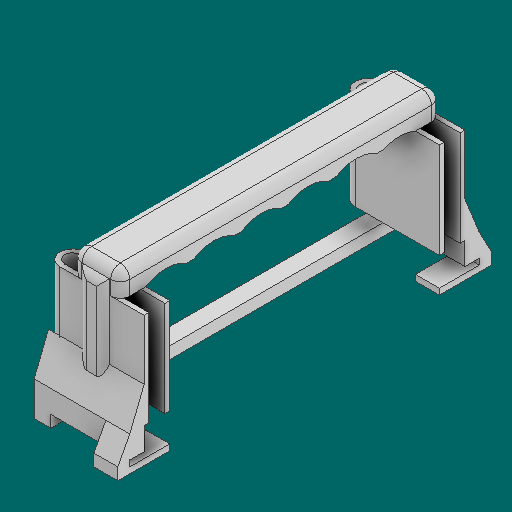
# Autodesk Inventor part: lab2
Saved by Autodesk Inventor 2026.1 (Build 301233000, 233)
## iProperties
Created: 2025-10-02
Part Number: lab2
Material: Genérico
Document SubType Name: Modeling
Designer: norbe
Density: 1 g/cm^3
Appearance: Valor por defecto
Author: norbe
Autodesk Inventor part; units mm, degrees
ref_plane "YZ Plane" through (0, 0, 0) normal (1, 0, 0) x (0, 1, 0)
ref_plane "XZ Plane" through (0, 0, 0) normal (0, 1, 0) x (-1, 0, 0)
sketch "Boceto1" plane through (0, 0, 0) normal (0, 1, 0) x (-1, 0, 0)
  line L0 (0, 0) -> (70.5, 0)
  line L1 (70.5, 0) -> (70.5, -135)
  line L2 (70.5, -135) -> (0, -135)
  line L3 (0, -135) -> (0, 0)
  line L4 (35.25, -64.3132) -> (35.25, -123.8882)
  line L5 (35.25, -125.8882) -> (35.25, -132.5882)
  arc A0 (35.25, -132.5882) -> (35.25, -125.8882) centre (35.25, -129.2382) ccw
  line L6 (0, -67.5) -> (7.0984, -67.5)
  arc A1 (35.25, -134.5882) -> (35.25, -123.8882) centre (35.25, -129.2382) ccw
  line L7 (35.25, -123.8882) -> (0, -123.8882)
  line L8 (35.25, -134.5882) -> (0, -134.5882)
  line L9 (35.25, -125.8882) -> (0, -125.8882)
  line L10 (35.25, -132.5882) -> (0, -132.5882)
  arc A2 (35.25, -11.1118) -> (35.25, -0.4118) centre (35.25, -5.7618) ccw
  line L11 (35.25, -11.1118) -> (0, -11.1118)
  line L12 (35.25, -0.4118) -> (0, -0.4118)
  arc A3 (35.25, -9.1118) -> (35.25, -2.4118) centre (35.25, -5.7618) ccw
  line L13 (35.25, -9.1118) -> (0, -9.1118)
  line L14 (35.25, -2.4118) -> (0, -2.4118)
  dimension "d0" = 70.5
  dimension "d1" = 135
  dimension "d2" = 61.575
  dimension "d3" = 6.7
  dimension "d4" = 67.5
  dimension "d5" = 2
  constraints: 30 end point, 10 symmetric about line, 8 point on circle, 4 centre point, 4 point on line, 3 horizontal, 3 parallel, 3 perpendicular, 2 midpoint, 2 tangent, 2 vertical, 2 other
  measures "d0" distance of L1.end L2.end
  measures "d1" distance of L0.end L1.end
  measures "d2" distance of L4.start L5.start
  measures "d3" distance of L5.end L5.start
  measures "d4" distance between parallel lines of L2 L6
  measures "d5" radial gap between concentric circles of A0 A1
extrude "Extrusión1" add sketch "Boceto1" along normal blind 40 contours L12 A2 L11 L3 L13 A3 L14 | L3 L10 A0 L9 L7 A1 L8
sketch "Boceto2" plane through (0, 0, -0.4118) normal (1, 0, 0) x (0, 0, -1)
  line L0 (0, 0) -> (2, 0) projected
  line L1 (2, 0) -> (2, 40) projected
  line L2 (0, 40) -> (2, 40) projected
  line L3 (0, 0) -> (0, 40) projected
  line L4 (132.1764, 0) -> (134.1764, 0) projected
  line L5 (134.1764, 0) -> (134.1764, 40) projected
  line L6 (132.1764, 40) -> (134.1764, 40) projected
  line L7 (132.1764, 0) -> (132.1764, 40) projected
  line L8 (0, 0) -> (134.1764, 0)
  line L9 (134.1764, 0) -> (134.1764, -9.4)
  line L10 (134.1764, -9.4) -> (0, -9.4)
  line L11 (0, -9.4) -> (0, 0)
  line L12 (134.1764, -9.4) -> (-1.655, -9.4)
  line L13 (-1.655, -9.4) -> (-1.655, -12.4)
  line L14 (-1.655, -12.4) -> (134.1764, -12.4)
  line L15 (134.1764, -12.4) -> (134.1764, -9.4)
  line L16 (134.1764, 0) -> (134.1764, 15)
  line L17 (134.1764, 0) -> (134.1764, 40) projected
  line L18 (134.1764, 0) -> (149.1764, 0) construction
  line L19 (134.1764, -9.4) -> (140.1764, -9.4)
  line L20 (140.1764, -9.4) -> (140.1764, 0)
  line L21 (134.1764, 15) -> (140.1764, 0)
  line L22 (67.0882, 0) -> (67.0882, 3.7714)
  line L23 (0, 0) -> (0, -9.4)
  line L24 (0, 0) -> (0, 15)
  line L25 (0, -9.4) -> (-6, -9.4)
  line L26 (-6, -9.4) -> (-6, 0)
  line L27 (0, 15) -> (-6, 0)
  point P0 (-0.4118, 0)
  point P1 (134.1764, 0)
  point P2 (0, -9.4)
  point P3 (0, -9.4)
  dimension "d8" = 9.4
  dimension "d9" = 3
  dimension "d19" = 15
  dimension "d20" = 90
  dimension "d21" = 6
  constraints: 38 end point, 4 horizontal, 4 parallel, 4 perpendicular, 4 symmetric about line, 1 collinear, 1 midpoint, 1 point on line, 1 vertical
  measures "d8" distance of L8.end L9.end
  measures "d9" distance of L13.end L12.end
  measures "d19" distance of L8.end L16.end
  measures "d20" angle of L18 L16
  measures "d21" distance of L9.end L19.end
extrude "Extrusión2" add sketch "Boceto2" against normal blind 40 contours L11 L12 L25 L26 L27 L3 | L0 L8 L4 L9 L10 L11 | L9 L5 L21 L20 L19
extrude "Extrusión3" add sketch "Boceto2" against normal blind 5 contours L10 L15 L14 L13 L12
sketch "Boceto4" plane through (-40, 0, -0.4118) normal (-1, 0, 0) x (0, 0, 1)
  line L0 (-134.1764, 15) -> (-140.1764, 0) projected
  line L1 (-140.1764, 0) -> (-140.1764, -9.4) projected
  line L2 (-140.1764, -9.4) -> (6, -9.4) projected
  line L3 (6, -9.4) -> (6, 0) projected
  line L4 (6, 0) -> (0, 15) projected
  line L5 (0, 15) -> (0, 0) projected
  line L6 (0, 0) -> (-2.8883, 0) projected
  line L7 (-7.8117, 0) -> (-2.8883, 0) projected
  line L8 (-7.8117, 0) -> (-126.3647, 0) projected
  line L9 (-131.2881, 0) -> (-126.3647, 0) projected
  line L10 (-131.2881, 0) -> (-134.1764, 0) projected
  line L11 (-134.1764, 0) -> (-134.1764, 15) projected
  line L12 (-140.1764, -9.4) -> (6, -9.4)
  line L13 (6, -9.4) -> (6, -14.4)
  line L14 (6, -14.4) -> (-140.1764, -14.4)
  line L15 (-140.1764, -14.4) -> (-140.1764, -9.4)
  line L16 (0, 0) -> (0, -9.4)
  line L17 (-134.1764, 0) -> (-134.1764, -9.4)
  point P0 (0.4118, 0)
  dimension "d22" = 5
  constraints: 12 end point, 3 perpendicular, 2 parallel, 2 point on line, 1 horizontal
  measures "d22" distance of L12.end L13.end
extrude "Extrusión4" cut sketch "Boceto4" against normal blind 40 contours L10 L9 L8 L7 L6 L16 L2 L17 | L2 L13 L14 L15
extrude "Extrusión5" add sketch "Boceto4" against normal blind 7 contours L2 L13 L14 L15
sketch "Boceto5" plane through (0, 0, -2.4118) normal (1, 0, 0) x (0, 0, -1)
  line L0 (-2, 40) -> (132.1764, 40)
  line L1 (132.1764, 40) -> (132.1764, 46)
  line L2 (128.1764, 50) -> (2, 50)
  line L3 (-2, 46) -> (-2, 40)
  arc A0 (25.7, 40) -> (8.7, 40) centre (17.2, 26.4446) ccw
  arc A1 (25.7, 40) -> (28.7, 40) centre (27.2, 44.7697) ccw
  line L4 (28.7, 40) -> (28.7, 41.5335)
  arc A2 (45.7, 40) -> (28.7, 40) centre (37.2, 26.4446) ccw
  arc A3 (45.7, 40) -> (48.7, 40) centre (47.2, 44.5587) ccw
  line L5 (48.7, 40) -> (48.7, 40.7668)
  arc A4 (65.7, 40) -> (48.7, 40) centre (57.2, 26.4446) ccw
  arc A5 (65.7, 40) -> (68.1808, 40) centre (66.9404, 43.0685) ccw
  arc A6 (85.1808, 40) -> (68.1808, 40) centre (76.6808, 26.4446) ccw
  arc A7 (85.1808, 40) -> (88.1808, 40) centre (86.6808, 44.5366) ccw
  arc A8 (105.1808, 40) -> (88.1808, 40) centre (96.6808, 26.4446) ccw
  arc A9 (105.1808, 40) -> (108.1808, 40) centre (106.6808, 42.3921) ccw
  arc A10 (121.4764, 40) -> (108.1808, 40) centre (114.8286, 25.4464) ccw
  arc A11 (2, 50) -> (-2, 46) centre (2, 46) ccw
  arc A12 (132.1764, 46) -> (128.1764, 50) centre (128.1764, 46) ccw
  point P0 (-2.4118, 0)
  point P1 (132.1764, 50)
  dimension "d27" = 10
  dimension "d28" = 17
  dimension "d29" = 16
  dimension "d30" = 5
  dimension "d31" = 3
  dimension "d32" = 17
  dimension "d33" = 16
  dimension "d39" = 3
  dimension "d40" = 17
  dimension "d41" = 16
  dimension "d42" = 17
  dimension "d43" = 16
  dimension "d44" = 3
  dimension "d45" = 17
  dimension "d46" = 16
  dimension "d47" = 3
  dimension "d48" = 16
  dimension "d49" = 4
  constraints: 26 point on circle, 13 centre point, 10 end point, 5 tangent, 3 vertical, 2 point on line, 1 coincident, 1 equal radius, 1 horizontal, 1 parallel, 13 other
  measures "d27" distance of point (132.176, 50) L1.start
  measures "d28" distance of A0.end A0.start
  measures "d29" radius of A0
  measures "d30" radius of A1
  measures "d31" distance of A0.start L4.start
  measures "d32" distance of L4.start A2.start
  measures "d33" radius of A2
  measures "d39" distance of A2.start L5.start
  measures "d40" distance of L5.start A4.start
  measures "d41" radius of A4
  measures "d42" distance of A5.end A6.start
  measures "d43" radius of A6
  measures "d44" distance of A6.start A7.end
  measures "d45" distance of A7.end A8.start
  measures "d46" radius of A8
  measures "d47" distance of A8.start A9.end
  measures "d48" radius of A10
  measures "d49" radius of A11
extrude "Extrusión6" add sketch "Boceto5" against normal blind 30 contours L3 A11 L2 A12 L1 L0 A10 A8 A6 A4 A2 A0
sketch "Boceto6" plane through (0, -9.4, -140.5882) normal (1, 0, 0) x (0, 0, -1)
  line L0 (-131.4764, 9.4) -> (-129.4764, 9.4) projected
  line L1 (-129.4764, 9.4) -> (-129.4764, 49.4) projected
  arc A0 (-112.4764, 49.4) -> (-129.4764, 49.4) centre (-120.9764, 35.8446) ccw projected
  line L2 (-112.4764, 49.4) -> (-109.4764, 49.4) projected
  arc A1 (-92.4764, 49.4) -> (-109.4764, 49.4) centre (-100.9764, 35.8446) ccw projected
  line L3 (-92.4764, 49.4) -> (-89.4764, 49.4) projected
  arc A2 (-72.4764, 49.4) -> (-89.4764, 49.4) centre (-80.9764, 35.8446) ccw projected
  line L4 (-72.4764, 49.4) -> (-69.9956, 49.4) projected
  arc A3 (-52.9956, 49.4) -> (-69.9956, 49.4) centre (-61.4956, 35.8446) ccw projected
  line L5 (-52.9956, 49.4) -> (-49.9956, 49.4) projected
  arc A4 (-32.9956, 49.4) -> (-49.9956, 49.4) centre (-41.4956, 35.8446) ccw projected
  line L6 (-32.9956, 49.4) -> (-29.9956, 49.4) projected
  arc A5 (-16.7, 49.4) -> (-29.9956, 49.4) centre (-23.3478, 34.8464) ccw projected
  line L7 (-16.7, 9.4) -> (-16.7, 49.4) projected
  line L8 (-16.7, 9.4) -> (-14.7, 9.4) projected
  line L9 (-14.7, 9.4) -> (-14.7, 49.4) projected
  line L10 (-14.7, 49.4) -> (-8, 49.4) projected
  line L11 (-8, 9.4) -> (-8, 49.4) projected
  line L12 (-8, 9.4) -> (-6, 9.4) projected
  line L13 (-6, 9.4) -> (-6, 0) projected
  line L14 (-6, 0) -> (0, 0) projected
  line L15 (0, 0) -> (0, 9.4) projected
  line L16 (0, 9.4) -> (-6, 24.4) projected
  line L17 (-6, 24.4) -> (-6, 55.4) projected
  arc A6 (-6, 55.4) -> (-10, 59.4) centre (-10, 55.4) ccw projected
  line L18 (-10, 59.4) -> (-136.1764, 59.4) projected
  arc A7 (-136.1764, 59.4) -> (-140.1764, 55.4) centre (-136.1764, 55.4) ccw projected
  line L19 (-140.1764, 24.4) -> (-140.1764, 55.4) projected
  line L20 (-140.1764, 24.4) -> (-146.1764, 9.4) projected
  line L21 (-146.1764, 9.4) -> (-146.1764, 0) projected
  line L22 (-146.1764, 0) -> (-140.1764, 0) projected
  line L23 (-140.1764, 0) -> (-140.1764, 9.4) projected
  line L24 (-140.1764, 9.4) -> (-138.1764, 9.4) projected
  line L25 (-138.1764, 9.4) -> (-138.1764, 49.4) projected
  line L26 (-138.1764, 49.4) -> (-131.4764, 49.4) projected
  line L27 (-131.4764, 9.4) -> (-131.4764, 49.4) projected
  line L28 (-6, 49.4) -> (-140.1764, 49.4)
  point P0 (-140.5882, 9.4)
  point P1 (-92.4764, 49.4)
  constraints: 1 point on line, 3 other
extrude "Extrusión7" cut sketch "Boceto6" against normal blind 10 contours L26 L28 L19 A7 L18 A6 L17 L10 A5 L6 A4 L5 A3 L4 A2 L3 A1 L2 A0
fillet "Empalme1" radius 4 10 edges at (-10, 48.8284, -133.4166) (-10, 43, -134.5882) (-10, 48.8284, -1.5834) (-10, 43, -0.4118) (-10, 50, -67.5) (-30, 48.8284, -133.4166) (-30, 43, -134.5882) (-30, 48.8284, -1.5834) (-30, 43, -0.4118) (-30, 50, -67.5)
ref_plane "Plano de trabajo1" through (-20, -9.4, -140.5882) normal (1, 0, 0) x (0, 0, -1)
sketch "Boceto7" plane through (-20, -9.4, -140.5882) normal (1, 0, 0) x (0, 0, -1)
  line L0 (-140.1764, 55.4) -> (-140.1764, 49.4) projected
  line L1 (-6, 49.4) -> (-6, 55.4) projected
  line L2 (-146.1764, 9.4) -> (-140.1764, 24.4) projected
  line L3 (-140.1764, 55.4) -> (-142.1764, 55.4)
  line L4 (-142.1764, 55.4) -> (-142.1764, 19.4)
  line L5 (-142.1764, 19.4) -> (-140.1764, 19.4)
  line L6 (-140.1764, 19.4) -> (-140.1764, 55.4)
  line L7 (-6, 55.4) -> (-4, 55.4)
  line L8 (-4, 55.4) -> (-4, 19.4)
  line L9 (-4, 19.4) -> (-6, 19.4)
  line L10 (-6, 19.4) -> (-6, 55.4)
  point P0 (-140.5882, 9.4)
  dimension "d55" = 2
  dimension "d56" = 2
  constraints: 16 end point, 4 parallel, 2 horizontal, 2 perpendicular, 2 point on line
  measures "d55" distance of L5.end L4.end
  measures "d56" distance of L8.end L9.end
extrude "Extrusión8" add sketch "Boceto7" along normal mid plane 11
fillet "Empalme2" radius 4 6 edges at (-20, 46, 1.5882) (-14.5, 28, 1.5882) (-25.5, 28, 1.5882) (-20, 46, -136.5882) (-14.5, 28, -136.5882) (-25.5, 28, -136.5882)
sketch "Boceto8" plane through (0, -9.4, 5.5882) normal (1, 0, 0) x (0, 0, -1)
  line L0 (8, 49.4) -> (6, 49.4) projected
  line L1 (6, 24.4) -> (6, 49.4) projected
  line L2 (6, 24.4) -> (0, 9.4) projected
  line L3 (0, 9.4) -> (0, 0) projected
  line L4 (0, 0) -> (6, 0) projected
  line L5 (6, 0) -> (6, 9.4) projected
  line L6 (6, 9.4) -> (8, 9.4) projected
  line L7 (8, 9.4) -> (8, 49.4) projected
  line L8 (140.1764, 49.4) -> (138.1764, 49.4) projected
  line L9 (138.1764, 9.4) -> (138.1764, 49.4) projected
  line L10 (138.1764, 9.4) -> (140.1764, 9.4) projected
  line L11 (140.1764, 9.4) -> (140.1764, 0) projected
  line L12 (140.1764, 0) -> (146.1764, 0) projected
  line L13 (146.1764, 0) -> (146.1764, 9.4) projected
  line L14 (146.1764, 9.4) -> (140.1764, 24.4) projected
  line L15 (140.1764, 24.4) -> (140.1764, 49.4) projected
  line L16 (140.1764, 9.4) -> (146.1764, 9.4)
  line L17 (140.1764, 0) -> (146.1764, 0) projected
  line L18 (6, 9.4) -> (0, 9.4)
  line L19 (146.1764, 0) -> (151.1764, 0)
  line L20 (151.1764, 0) -> (151.1764, -5)
  line L21 (151.1764, -5) -> (129.4764, -5)
  line L22 (129.4764, -5) -> (129.4764, -2.5)
  line L23 (129.4764, -2.5) -> (151.1764, -2.5)
  line L24 (146.1764, 0) -> (146.1764, -2.5)
  line L25 (0, -5) -> (146.1764, -5) projected
  line L26 (73.0882, -5) -> (73.0882, -8.447)
  line L27 (0, 0) -> (-5, 0)
  line L28 (-5, 0) -> (-5, -5)
  line L29 (-5, -5) -> (16.7, -5)
  line L30 (16.7, -2.5) -> (-5, -2.5)
  line L31 (0, 0) -> (0, -2.5)
  line L32 (16.7, -2.5) -> (16.7, -5)
  line L33 (0, 9.4) -> (0, 0) projected
  line L34 (-5, 0) -> (0, 9.4)
  line L35 (151.1764, 0) -> (146.1764, 9.4)
  point P0 (5.5882, 9.4)
  dimension "d60" = 5
  constraints: 34 end point, 6 symmetric about line, 5 perpendicular, 3 point on line, 2 midpoint, 1 horizontal, 1 parallel, 1 vertical
  measures "d60" distance of L12.end L19.end
extrude "Extrusión9" add sketch "Boceto8" against normal blind 10 contours L3 L27 L34 | L31 L30 L28 L27 | L30 L32 L25 L29 L28 | L35 L19 L13 | L19 L20 L23 L24 | L23 L20 L21 L22
equation "\"d4\" = 0.5 * d1"
